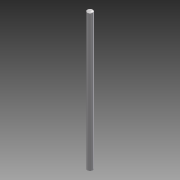
# Autodesk Inventor part: shaft
Saved by Autodesk Inventor 2016 (Build 200138000, 138)
## iProperties
Created: 2014-07-17
Part Number: shaft
Material: Steel, Cast
Document SubType Name: Modeling
Designer: Sebastian
Density: 7.85 g/cm^3
Appearance: Semi-Polished
Mass: 4.16132 g
Surface Area: 7.20178 cm^2
Volume: 0.530104 cm^3
Author: Sebastian
Autodesk Inventor part; units mm, degrees
ref_plane "YZ Plane" through (0, 0, 0) normal (1, 0, 0) x (0, 1, 0)
ref_plane "XZ Plane" through (0, 0, 0) normal (0, 1, 0) x (-1, 0, 0)
ref_plane "XY Plane" through (0, 0, 0) normal (0, 0, 1) x (1, 0, 0)
sketch "Sketch1" plane through (0, 0, 0) normal (0, 0, 1) x (1, 0, 0)
  circle A0 centre (0, 0) radius 1.5
  dimension "d0" = 3
  constraints: 1 centre point, 1 coincident
  measures "d0" diameter of A0
extrude "Extrusion1" add sketch "Sketch1" along normal blind 75
fillet "Fillet1" radius 0.1 2 edges at (-1.5, 0, 75) (-1.5, 0, 0)
body "Solid1"
